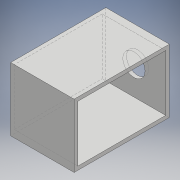
# Autodesk Inventor part: 車軸受け2
Saved by Autodesk Inventor 2018 (Build 220112000, 112)
## iProperties
Created: 2017-09-15
Part Number: 車軸受け2
Material: 一般
Document SubType Name: Modeling
Designer: mura5
Density: 1 g/cm^3
Appearance: 既定
Author: mura5
Autodesk Inventor part; units mm, degrees
ref_plane "YZ Plane" through (0, 0, 0) normal (1, 0, 0) x (0, 1, 0)
ref_plane "XZ Plane" through (0, 0, 0) normal (0, 1, 0) x (-1, 0, 0)
ref_plane "XY Plane" through (0, 0, 0) normal (0, 0, 1) x (1, 0, 0)
sketch "スケッチ1" plane through (0, 0, 0) normal (1, 0, 0) x (0, 1, 0)
  line L0 (-30, 20) -> (30, 20)
  line L1 (30, 20) -> (30, -20)
  line L2 (30, -20) -> (-30, -20)
  line L3 (-30, -20) -> (-30, 20)
  line L4 (-30, 20) -> (30, -20) construction
  line L5 (30, 20) -> (-30, -20) construction
  line L6 (27.7, -17.7) -> (27.7, 17.7)
  line L7 (27.7, 17.7) -> (-27.7, 17.7)
  line L8 (-27.7, 17.7) -> (-27.7, -17.7)
  line L9 (-27.7, -17.7) -> (27.7, -17.7)
  point P0 (0, 0)
  dimension "d0" = 60
  dimension "d1" = 40
  dimension "d2" = 2.3
  constraints: 20 end point, 4 parallel, 2 midpoint, 2 perpendicular, 1 horizontal, 3 other
  measures "d0" distance of L1.end L2.end
  measures "d1" distance of L0.end L1.end
  measures "d2" distance between parallel lines of L1 L6
extrude "押し出し1" add sketch "スケッチ1" along normal mid plane 40
sketch "スケッチ2" plane through (-20, 30, 20) normal (0, 1, 0) x (1, 0, 0)
  line L0 (0, 0) -> (0, 40) projected
  circle A0 centre (20, 20) radius 7
  dimension "d6" = 14
  dimension "d7" = 20
  constraints: 1 centre point
  measures "d6" diameter of A0
  measures "d7" distance from line of L0 A0.centre
extrude "押し出し2" cut sketch "スケッチ2" against normal blind 5
